TEST generated POWER BOX  6 CUT first showing drilling in contour_v3 (Autodesk Fusion 360 design; units mm, degrees)
Autodesk Fusion 360 part; units mm, degrees
sketch "b  stock" plane through (0, 0, 0) normal (0, 0, 1) x (1, 0, 0)
  line L0 (0, 0) -> (304.8, 0)
  line L1 (304.8, 0) -> (304.8, 609.6)
  line L2 (304.8, 609.6) -> (0, 609.6)
  line L3 (0, 609.6) -> (0, 0)
extrude "b  stock body extrude Feature" add sketch "b  stock" along normal blind 3.175 makes body 1
sketch "b  layout" plane through (0, 0, 0) normal (0, 0, 1) x (1, 0, 0)
  line L0 (0, 0) -> (90, 0)
  line L1 (90, 0) -> (90, 85)
  line L2 (90, 85) -> (0, 85)
  line L3 (0, 85) -> (0, 0)
  line L4 (92.01, 0) -> (182.01, 0)
  line L5 (182.01, 0) -> (182.01, 85)
  line L6 (182.01, 85) -> (92.01, 85)
  line L7 (92.01, 85) -> (92.01, 0)
  line L8 (184.02, 0) -> (234.02, 0)
  line L9 (234.02, 0) -> (234.02, 85)
  line L10 (234.02, 85) -> (184.02, 85)
  line L11 (184.02, 85) -> (184.02, 0)
  line L12 (236.03, 0) -> (286.03, 0)
  line L13 (286.03, 0) -> (286.03, 85)
  line L14 (286.03, 85) -> (236.03, 85)
  line L15 (236.03, 85) -> (236.03, 0)
  line L16 (0, 87.01) -> (90, 87.01)
  line L17 (90, 87.01) -> (90, 137.01)
  line L18 (90, 137.01) -> (0, 137.01)
  line L19 (0, 137.01) -> (0, 87.01)
  line L20 (92.01, 87.01) -> (182.01, 87.01)
  line L21 (182.01, 87.01) -> (182.01, 137.01)
  line L22 (182.01, 137.01) -> (92.01, 137.01)
  line L23 (92.01, 137.01) -> (92.01, 87.01)
sketch "b top lines" plane through (0, 0, 0) normal (0, 0, 1) x (1, 0, 0)
  line L0 (0, 0) -> (10.15, 0)
  line L1 (10.15, 0) -> (10.15, 3.175)
  line L2 (10.15, 3.175) -> (19.85, 3.175)
  line L3 (19.85, 3.175) -> (19.85, 0)
  line L4 (19.85, 0) -> (30.15, 0)
  line L5 (30.15, 0) -> (30.15, 3.175)
  line L6 (30.15, 3.175) -> (39.85, 3.175)
  line L7 (39.85, 3.175) -> (39.85, 0)
  line L8 (39.85, 0) -> (50.15, 0)
  line L9 (50.15, 0) -> (50.15, 3.175)
  line L10 (50.15, 3.175) -> (59.85, 3.175)
  line L11 (59.85, 3.175) -> (59.85, 0)
  line L12 (59.85, 0) -> (70.15, 0)
  line L13 (70.15, 0) -> (70.15, 3.175)
  line L14 (70.15, 3.175) -> (79.85, 3.175)
  line L15 (79.85, 3.175) -> (79.85, 0)
  line L16 (79.85, 0) -> (90, 0)
  line L17 (90, 0) -> (90, 17.65)
  line L18 (90, 17.65) -> (86.825, 17.65)
  line L19 (86.825, 17.65) -> (86.825, 27.35)
  line L20 (86.825, 27.35) -> (90, 27.35)
  line L21 (90, 27.35) -> (90, 37.65)
  line L22 (90, 37.65) -> (86.825, 37.65)
  line L23 (86.825, 37.65) -> (86.825, 47.35)
  line L24 (86.825, 47.35) -> (90, 47.35)
  line L25 (90, 47.35) -> (90, 57.65)
  line L26 (90, 57.65) -> (86.825, 57.65)
  line L27 (86.825, 57.65) -> (86.825, 67.35)
  line L28 (86.825, 67.35) -> (90, 67.35)
  line L29 (90, 67.35) -> (90, 85)
  line L30 (0, 85) -> (10.15, 85)
  line L31 (10.15, 85) -> (10.15, 81.825)
  line L32 (10.15, 81.825) -> (19.85, 81.825)
  line L33 (19.85, 81.825) -> (19.85, 85)
  line L34 (19.85, 85) -> (30.15, 85)
  line L35 (30.15, 85) -> (30.15, 81.825)
  line L36 (30.15, 81.825) -> (39.85, 81.825)
  line L37 (39.85, 81.825) -> (39.85, 85)
  line L38 (39.85, 85) -> (50.15, 85)
  line L39 (50.15, 85) -> (50.15, 81.825)
  line L40 (50.15, 81.825) -> (59.85, 81.825)
  line L41 (59.85, 81.825) -> (59.85, 85)
  line L42 (59.85, 85) -> (70.15, 85)
  line L43 (70.15, 85) -> (70.15, 81.825)
  line L44 (70.15, 81.825) -> (79.85, 81.825)
  line L45 (79.85, 81.825) -> (79.85, 85)
  line L46 (79.85, 85) -> (90, 85)
  line L47 (0, 0) -> (0, 17.65)
  line L48 (0, 17.65) -> (3.175, 17.65)
  line L49 (3.175, 17.65) -> (3.175, 27.35)
  line L50 (3.175, 27.35) -> (0, 27.35)
  line L51 (0, 27.35) -> (0, 37.65)
  line L52 (0, 37.65) -> (3.175, 37.65)
  line L53 (3.175, 37.65) -> (3.175, 47.35)
  line L54 (3.175, 47.35) -> (0, 47.35)
  line L55 (0, 47.35) -> (0, 57.65)
  line L56 (0, 57.65) -> (3.175, 57.65)
  line L57 (3.175, 57.65) -> (3.175, 67.35)
  line L58 (3.175, 67.35) -> (0, 67.35)
  line L59 (0, 67.35) -> (0, 85)
sketch "b top circles" plane through (0, 0, 0) normal (0, 0, 1) x (1, 0, 0)
  circle A0 centre (10.6806, 2.4644) radius 1.005
  circle A1 centre (19.3194, 2.4644) radius 1.005
  circle A2 centre (30.6806, 2.4644) radius 1.005
  circle A3 centre (39.3194, 2.4644) radius 1.005
  circle A4 centre (50.6806, 2.4644) radius 1.005
  circle A5 centre (59.3194, 2.4644) radius 1.005
  circle A6 centre (70.6806, 2.4644) radius 1.005
  circle A7 centre (79.3194, 2.4644) radius 1.005
  circle A8 centre (87.5356, 18.1806) radius 1.005
  circle A9 centre (87.5356, 26.8194) radius 1.005
  circle A10 centre (87.5356, 38.1806) radius 1.005
  circle A11 centre (87.5356, 46.8194) radius 1.005
  circle A12 centre (87.5356, 58.1806) radius 1.005
  circle A13 centre (87.5356, 66.8194) radius 1.005
  circle A14 centre (10.6806, 82.5356) radius 1.005
  circle A15 centre (19.3194, 82.5356) radius 1.005
  circle A16 centre (30.6806, 82.5356) radius 1.005
  circle A17 centre (39.3194, 82.5356) radius 1.005
  circle A18 centre (50.6806, 82.5356) radius 1.005
  circle A19 centre (59.3194, 82.5356) radius 1.005
  circle A20 centre (70.6806, 82.5356) radius 1.005
  circle A21 centre (79.3194, 82.5356) radius 1.005
  circle A22 centre (2.4644, 18.1806) radius 1.005
  circle A23 centre (2.4644, 26.8194) radius 1.005
  circle A24 centre (2.4644, 38.1806) radius 1.005
  circle A25 centre (2.4644, 46.8194) radius 1.005
  circle A26 centre (2.4644, 58.1806) radius 1.005
  circle A27 centre (2.4644, 66.8194) radius 1.005
extrude "b top lines lines extrude Feature" add sketch "b top lines" along normal blind 3.175 separate body makes body 2
extrude "b top circles circles extrude Feature" add sketch "b top circles" along normal blind 3.175 separate body makes body 3 at (3.4644, 58.0806, 2.1167) makes body 4 at (3.4644, 38.0806, 2.1167) makes body 5 at (3.4644, 18.0806, 2.1167) makes body 6 at (69.7363, 82.8794, 2.1167) makes body 7 at (49.7363, 82.8794, 2.1167) makes body 8 at (31.6067, 82.926, 2.1167) makes body 9 at (9.7363, 82.8794, 2.1167) makes body 10 at (86.5913, 67.1631, 2.1167) makes body 11 at (87.2156, 45.8667, 1.0583) makes body 12 at (87.2156, 25.8667, 1.0583) makes body 13 at (78.9993, 1.5117, 1.0583) makes body 14 at (59.2943, 3.469, 2.1167) makes body 15 at (39.2943, 3.469, 2.1167) makes body 16 at (20.3194, 2.3643, 2.1167) makes body 17 at (31.6806, 2.3643, 2.1167) makes body 18 at (50.6556, 3.469, 2.1167) makes body 19 at (70.3606, 1.5117, 1.0583) makes body 20 at (87.2156, 17.228, 1.0583) makes body 21 at (87.2156, 37.228, 1.0583) makes body 22 at (87.2156, 57.228, 1.0583) makes body 23 at (11.6806, 2.3643, 2.1167) makes body 24 at (20.2454, 82.926, 2.1167) makes body 25 at (38.375, 82.8794, 2.1167) makes body 26 at (58.375, 82.8794, 2.1167) makes body 27 at (78.375, 82.8794, 2.1167) makes body 28 at (3.4644, 26.7193, 2.1167) makes body 29 at (3.4644, 46.7193, 2.1167) makes body 30 at (3.3904, 67.2097, 2.1167)
combine "b top lines final combine feature" operation cut target body 2 tool bodies 3 4 5 6 7 8 9 10 11 12 13 14 15 16 17 18 19 20 21 22 23 24 25 26 27 28 29 30
equation "d1163 = length"
equation "d1817 = depth"
equation "d289 = platformGrommetMountDiameter"
equation "d422 = length"
equation "d423 = depth"
equation "d843 = toolDiameter"
equation "d1634 = pcbMountHoles"
equation "d1797 = ( depth - 26 mm ) / 2"
equation "d1798 = ( length - 58 mm ) / 2"
equation "d492 = length"
equation "d493 = height"
equation "d502 = length"
equation "d503 = height"
equation "d1827 = depth"
equation "d1829 = ventDiameter"
equation "d910 = depth"
equation "d911 = height"
equation "d1819 = ventDiameter"
equation "b_ = 5 mm" comment "added by script"
named bodies: "b  stockbody", "b top lines final body", "b top circles circle body", "b top circles circle body (1)", "b top circles circle body (2)", "b top circles circle body (3)", "b top circles circle body (4)", "b top circles circle body (5)", "b top circles circle body (6)", "b top circles circle body (7)", "b top circles circle body (8)", "b top circles circle body (9)", "b top circles circle body (10)", "b top circles circle body (11)", "b top circles circle body (12)", "b top circles circle body (13)", "b top circles circle body (14)", "b top circles circle body (15)", "b top circles circle body (16)", "b top circles circle body (17)", "b top circles circle body (18)", "b top circles circle body (19)", "b top circles circle body (20)", "b top circles circle body (21)", "b top circles circle body (22)", "b top circles circle body (23)", "b top circles circle body (24)", "b top circles circle body (25)", "b top circles circle body (26)", "b top circles circle body (27)"
